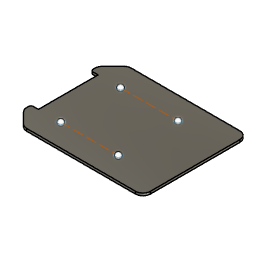
MicroMouse_PCB v8 (Autodesk Fusion 360 design; units mm, degrees)
Autodesk Fusion 360 part; units mm, degrees
sketch "Sketch1" plane through (0, 0, 0) normal (0, 0, 1) x (1, 0, 0)
  line L0 (45, -35) -> (-45, -35)
  line L1 (-45, -35) -> (-45, 35)
  line L2 (-45, 35) -> (45, 35)
  line L3 (45, 35) -> (45, -35)
  line L4 (45, -35) -> (-45, 35) construction
  line L5 (-45, -35) -> (45, 35) construction
  dimension "d1" = 90
  dimension "d2" = 70
  constraint horizontal L0
  constraint perpendicular L0 L1
  constraint parallel L0 L2
  constraint parallel L1 L3
  constraint coincident L4 origin
  constraint coincident L5 origin
  measures "d1" distance of L1.end L2.end
  measures "d2" distance of L0.end L1.end
extrude "Extrude1" add sketch "Sketch1" along normal blind 1.6
fillet "Fillet1" radius 5 2 edges at (45, -35, 0.8) (45, 35, 0.8)
chamfer "Chamfer1" distance 10 angle 45 2 edges at (-45, -35, 0.8) (-45, 35, 0.8)
fillet "Fillet2" radius 5 4 edges at (-35, 35, 0.8) (-45, 25, 0.8) (-45, -25, 0.8) (-35, -35, 0.8)
sketch "Sketch2" plane through (0, 0, 1.6) normal (0, 0, 1) x (-1, 0, 0)
  arc A0 (36.4645, 33.5355) -> (32.9289, 35) centre (32.9289, 30) ccw
  line L0 (32.9289, 35) -> (-40, 35)
  arc A1 (-40, 35) -> (-45, 30) centre (-40, 30) ccw
  line L1 (-45, 30) -> (-45, -30)
  arc A2 (-45, -30) -> (-40, -35) centre (-40, -30) ccw
  line L2 (-40, -35) -> (32.9289, -35)
  arc A3 (32.9289, -35) -> (36.4645, -33.5355) centre (32.9289, -30) ccw
  line L3 (36.4645, -33.5355) -> (43.5355, -26.4645)
  arc A4 (43.5355, -26.4645) -> (45, -22.9289) centre (40, -22.9289) ccw
  line L4 (45, -22.9289) -> (45, 22.9289)
  arc A5 (45, 22.9289) -> (43.5355, 26.4645) centre (40, 22.9289) ccw
  line L5 (43.5355, 26.4645) -> (36.4645, 33.5355)
  line L6 (-25, -20) -> (25, -20)
  line L7 (25, -20) -> (25, 20)
  line L8 (25, 20) -> (-25, 20)
  line L9 (-25, 20) -> (-25, -20)
  line L10 (-25, -20) -> (25, 20) construction
  line L11 (25, -20) -> (-25, 20) construction
  circle A6 centre (25, 20) radius 1.75
  circle A7 centre (25, -20) radius 1.75
  dimension "d10" = 50
  dimension "d11" = 40
  dimension "d12" = 3.5
  dimension "d13" = 3.5
  constraint horizontal L6
  constraint perpendicular L6 L7
  constraint parallel L6 L8
  constraint parallel L7 L9
  constraint coincident L10 origin
  constraint coincident L11 origin
  constraint coincident L7.end L8.start
  constraint coincident L6.end L7.start
  measures "d10" distance of L7.end L8.end
  measures "d11" distance of L6.end L7.end
  measures "d12" diameter of A6
  measures "d13" diameter of A7
sketch "Sketch16" plane through (0, 0, 1.6) normal (0, 0, 1) x (-1, 0, 0)
  line L0 (25, 20) -> (-13.5, 20) construction
  line L1 (25, -20) -> (-13.5, -20) construction
  dimension "d32" = 38.5
  dimension "d33" = 38.5
  constraint horizontal L0
  constraint horizontal L1
  measures "d32" distance of L0.start L0.end
  measures "d33" distance of L1.start L1.end
sketch "Sketch17" plane through (0, 0, 1.6) normal (0, 0, 1) x (1, 0, 0)
  circle A0 centre (-25, 20) radius 1.8
  circle A1 centre (13.5, 20) radius 1.8
  circle A2 centre (-25, -20) radius 1.8
  circle A3 centre (13.5, -20) radius 1.8
  dimension "d34" = 3.6
  dimension "d35" = 3.6
  dimension "d36" = 3.6
  dimension "d37" = 3.6
  measures "d34" diameter of A0
  measures "d35" diameter of A1
  measures "d36" diameter of A2
  measures "d37" diameter of A3
extrude "Extrude7" cut sketch "Sketch17" against normal blind 4 contours A2
extrude "Extrude8" cut sketch "Sketch17" against normal blind 5 contours A3
extrude "Extrude9" cut sketch "Sketch17" against normal blind 4 contours A1
extrude "Extrude10" cut sketch "Sketch17" against normal blind 65 contours A0
sketch "Sketch18" plane through (0, 0, 1.6) normal (0, 0, 1) x (-1, 0, 0)
  circle A0 centre (25, -20) radius 1.8
  circle A1 centre (-13.5, -20) radius 1.8
  circle A2 centre (-13.5, 20) radius 1.8
  circle A3 centre (25, 20) radius 1.8
  arc A4 (36.4645, 33.5355) -> (32.9289, 35) centre (32.9289, 30) ccw
  line L0 (32.9289, 35) -> (-40, 35)
  arc A5 (-40, 35) -> (-45, 30) centre (-40, 30) ccw
  line L1 (-45, 30) -> (-45, -30)
  arc A6 (-45, -30) -> (-40, -35) centre (-40, -30) ccw
  line L2 (-40, -35) -> (32.9289, -35)
  arc A7 (32.9289, -35) -> (36.4645, -33.5355) centre (32.9289, -30) ccw
  line L3 (36.4645, -33.5355) -> (43.5355, -26.4645)
  arc A8 (43.5355, -26.4645) -> (45, -22.9289) centre (40, -22.9289) ccw
  line L4 (45, -22.9289) -> (45, 22.9289)
  arc A9 (45, 22.9289) -> (43.5355, 26.4645) centre (40, 22.9289) ccw
  line L5 (43.5355, 26.4645) -> (36.4645, 33.5355)
  line L6 (40, 20) -> (50, 20)
  line L7 (50, 20) -> (50, -20)
  line L8 (50, -20) -> (40, -20)
  line L9 (40, -20) -> (40, 20)
  line L10 (40, 20) -> (50, -20) construction
  line L11 (50, 20) -> (40, -20) construction
  point P0 (45, 0)
  dimension "d46" = 10
  constraint horizontal L6
  constraint perpendicular L6 L7
  constraint parallel L6 L8
  constraint parallel L7 L9
  constraint coincident L10 P0
  constraint coincident L11 P0
  constraint midpoint L4 P0
  measures "d46" distance of L7.end L8.end
extrude "Extrude11" cut sketch "Sketch18" against normal blind 100 contours L4 L6 L8 L9
chamfer "Chamfer4" distance 1 angle 45 2 edges at (-45, 20, 0.8) (-45, -20, 0.8)
extrude "Extrude2" [suppressed]
sketch "Sketch3" plane through (0, 0, 1.6) normal (0, 0, 1) x (-1, 0, 0)
  arc A0 (36.4645, 33.5355) -> (32.9289, 35) centre (32.9289, 30) ccw
  line L0 (32.9289, 35) -> (-40, 35)
  arc A1 (-40, 35) -> (-45, 30) centre (-40, 30) ccw
  line L1 (-45, 30) -> (-45, -30)
  arc A2 (-45, -30) -> (-40, -35) centre (-40, -30) ccw
  line L2 (-40, -35) -> (32.9289, -35)
  arc A3 (32.9289, -35) -> (36.4645, -33.5355) centre (32.9289, -30) ccw
  line L3 (36.4645, -33.5355) -> (43.5355, -26.4645)
  arc A4 (43.5355, -26.4645) -> (45, -22.9289) centre (40, -22.9289) ccw
  line L4 (45, -22.9289) -> (45, 22.9289)
  arc A5 (45, 22.9289) -> (43.5355, 26.4645) centre (40, 22.9289) ccw
  line L5 (43.5355, 26.4645) -> (36.4645, 33.5355)
  line L6 (40, -20) -> (50, -20)
  line L7 (50, -20) -> (50, 20)
  line L8 (50, 20) -> (40, 20)
  line L9 (40, 20) -> (40, -20)
  line L10 (40, -20) -> (50, 20) construction
  line L11 (50, -20) -> (40, 20) construction
  line L12 (-25, 20) -> (23.25, 20)
  arc A6 (25, 18.25) -> (23.25, 20) centre (25, 20) ccw
  line L13 (25, 18.25) -> (25, -18.25)
  arc A7 (23.25, -20) -> (25, -18.25) centre (25, -20) ccw
  line L14 (23.25, -20) -> (-25, -20)
  line L15 (-25, -20) -> (-25, 20)
  point P0 (45, 0)
  constraint horizontal L6
  constraint perpendicular L6 L7
  constraint parallel L6 L8
  constraint parallel L7 L9
  constraint coincident L10 P0
  constraint coincident L11 P0
  constraint midpoint L4 P0
extrude "Extrude3" [suppressed]
chamfer "Chamfer2" [suppressed]
chamfer "Chamfer3" [suppressed]
sketch "Sketch4" plane through (0, 0, 1.6) normal (0, 0, 1) x (-1, 0, 0)
  line L0 (45, -21) -> (44, -20)
  line L1 (44, -20) -> (40, -20)
  line L2 (40, -20) -> (40, 20)
  line L3 (40, 20) -> (44, 20)
  line L4 (44, 20) -> (45, 21)
  line L5 (45, 21) -> (45, 22.9289)
  arc A0 (45, 22.9289) -> (43.5355, 26.4645) centre (40, 22.9289) ccw
  line L6 (43.5355, 26.4645) -> (36.4645, 33.5355)
  arc A1 (36.4645, 33.5355) -> (32.9289, 35) centre (32.9289, 30) ccw
  line L7 (32.9289, 35) -> (-40, 35)
  arc A2 (-40, 35) -> (-45, 30) centre (-40, 30) ccw
  line L8 (-45, 30) -> (-45, -30)
  arc A3 (-45, -30) -> (-40, -35) centre (-40, -30) ccw
  line L9 (-40, -35) -> (32.9289, -35)
  arc A4 (32.9289, -35) -> (36.4645, -33.5355) centre (32.9289, -30) ccw
  line L10 (36.4645, -33.5355) -> (43.5355, -26.4645)
  arc A5 (43.5355, -26.4645) -> (45, -22.9289) centre (40, -22.9289) ccw
  line L11 (45, -22.9289) -> (45, -21)
  line L12 (-25, 20) -> (23.25, 20)
  arc A6 (25, 18.25) -> (23.25, 20) centre (25, 20) ccw
  line L13 (25, 18.25) -> (25, -18.25)
  arc A7 (23.25, -20) -> (25, -18.25) centre (25, -20) ccw
  line L14 (23.25, -20) -> (-25, -20)
  line L15 (-25, -20) -> (-25, 20)
sketch "Sketch5" plane through (0, 0, 1.6) normal (0, 0, 1) x (-1, 0, 0)
sketch "Sketch6" plane through (0, 0, 1.6) normal (0, 0, 1) x (-1, 0, 0)
sketch "Sketch7" plane through (0, 0, 1.6) normal (0, 0, 1) x (-1, 0, 0)
  line L0 (-45, -20) -> (-13.5, -20) construction
  dimension "d22" = 31.5
  constraint horizontal L0
  measures "d22" distance of L0.start L0.end
sketch "Sketch8" plane through (0, 0, 1.6) normal (0, 0, 1) x (-1, 0, 0)
  circle A0 centre (-13.5, -20) radius 1.8
  dimension "d23" = 3.6
  measures "d23" diameter of A0
sketch "Sketch9" plane through (0, 0, 1.6) normal (0, 0, 1) x (-1, 0, 0)
  line L0 (-45, 20) -> (-13.5, 20) construction
  dimension "d24" = 31.5
  constraint horizontal L0
  measures "d24" distance of L0.start L0.end
sketch "Sketch10" plane through (0, 0, 1.6) normal (0, 0, 1) x (-1, 0, 0)
  circle A0 centre (-13.5, 20) radius 1.8
  dimension "d25" = 3.6
  measures "d25" diameter of A0
extrude "Extrude4" [suppressed]
sketch "Sketch11" plane through (0, 0, 1.6) normal (0, 0, 1) x (-1, 0, 0)
  line L0 (45, -21) -> (44, -20)
  line L1 (44, -20) -> (40, -20)
  line L2 (40, -20) -> (40, 20)
  line L3 (40, 20) -> (44, 20)
  line L4 (44, 20) -> (45, 21)
  line L5 (45, 21) -> (45, 22.9289)
  arc A0 (45, 22.9289) -> (43.5355, 26.4645) centre (40, 22.9289) ccw
  line L6 (43.5355, 26.4645) -> (36.4645, 33.5355)
  arc A1 (36.4645, 33.5355) -> (32.9289, 35) centre (32.9289, 30) ccw
  line L7 (32.9289, 35) -> (-40, 35)
  arc A2 (-40, 35) -> (-45, 30) centre (-40, 30) ccw
  line L8 (-45, 30) -> (-45, -30)
  arc A3 (-45, -30) -> (-40, -35) centre (-40, -30) ccw
  line L9 (-40, -35) -> (32.9289, -35)
  arc A4 (32.9289, -35) -> (36.4645, -33.5355) centre (32.9289, -30) ccw
  line L10 (36.4645, -33.5355) -> (43.5355, -26.4645)
  arc A5 (43.5355, -26.4645) -> (45, -22.9289) centre (40, -22.9289) ccw
  line L11 (45, -22.9289) -> (45, -21)
  line L12 (-25, -20) -> (-2.3042, 31.9513) construction
  arc A6 (-15.3, -20) -> (-11.7, -20) centre (-13.5, -20) ccw
  line L13 (-15.3, -20) -> (-25, -20)
  line L14 (-25, -20) -> (-25, 20)
  line L15 (-25, 20) -> (-15.3, 20)
  arc A7 (-11.7, 20) -> (-15.3, 20) centre (-13.5, 20) ccw
  line L16 (-11.7, 20) -> (23.25, 20)
  arc A8 (25, 18.25) -> (23.25, 20) centre (25, 20) ccw
  line L17 (25, 18.25) -> (25, -18.25)
  arc A9 (23.25, -20) -> (25, -18.25) centre (25, -20) ccw
  line L18 (23.25, -20) -> (-11.7, -20)
sketch "Sketch12" plane through (0, 0, 1.6) normal (0, 0, 1) x (-1, 0, 0)
  line L0 (-13.5111, -20.0267) -> (-13.5111, -35)
  line L1 (-13.5111, -35) -> (-13.5111, -20.0267)
  constraint vertical L0
extrude "Extrude5" [suppressed]
extrude "Extrude6" [suppressed]
sketch "Sketch13" plane through (0, 0, 1.6) normal (0, 0, 1) x (-1, 0, 0)
  line L0 (25, 20) -> (-25, 20)
  constraint horizontal L0
sketch "Sketch14" plane through (0, 0, 1.6) normal (0, 0, 1) x (-1, 0, 0)
  line L0 (25, 20) -> (-25, 20) construction
  constraint horizontal L0
sketch "Sketch15" plane through (0, 0, 1.6) normal (0, 0, 1) x (-1, 0, 0)
  line L0 (25, 20) -> (-14, 20) construction
  line L1 (-14, 20) -> (-44, 9) construction
  constraint horizontal L0
